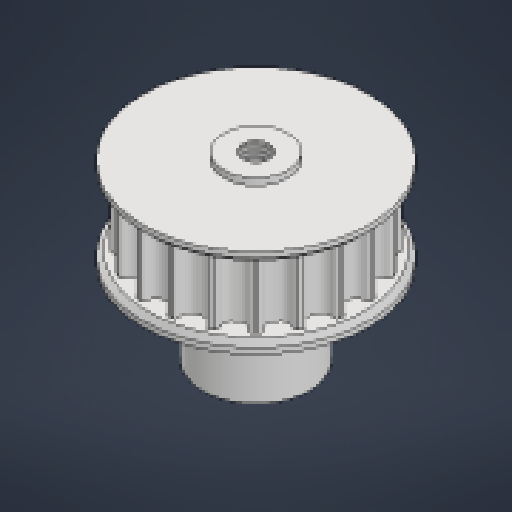
# Autodesk Inventor part: 3DPRINT,ROLLER,PLUG,SHORT
Saved by Autodesk Inventor 2026.1 (Build 301233020, 233B)
## iProperties
Created: 2026-03-30
Part Number: 3DPRINT,ROLLER,PLUG,SHORT
Material: Generic
Document SubType Name: Modeling
Designer: Owen L
Density: 1 g/cm^3
Appearance: Default
Author: Owen L
Autodesk Inventor part; units mm, degrees
(part 1 of 2)
ref_plane "YZ Plane" through (0, 0, 0) normal (1, 0, 0) x (0, 1, 0)
ref_plane "XZ Plane" through (0, 0, 0) normal (0, 1, 0) x (-1, 0, 0)
ref_plane "XY Plane" through (0, 0, 0) normal (0, 0, 1) x (1, 0, 0)
sketch "Sketch1" plane through (0, 0, 0) normal (0, 1, 0) x (-1, 0, 0)
  arc A0 (15.108, -2.6737) -> (15.1947, -2.1258) centre (0, 0) ccw
  spline S0 degree 3 poles (15.108, -2.6737) (15.0887, -2.737) (15.0572, -2.7959) (14.9734, -2.8984) (14.922, -2.941) (14.8056, -3.0039) (14.7419, -3.0237) (14.6027, -3.0386) (14.545, -3.0287) (14.2674, -2.9716) (14.0596, -2.9092) (13.6157, -2.9838) (13.4596, -3.0427) (13.1787, -3.2171) (13.0566, -3.3308) (12.8434, -3.6259) (12.7944, -3.773) (12.6632, -4.1825) (12.5425, -4.4508) (12.5133, -4.8985) (12.5344, -5.0632) (12.6389, -5.3764) (12.7214, -5.5216) (12.91, -5.7403) (13.0253, -5.8538) (13.397, -6.0406) (13.5567, -6.0705) (13.7265, -6.2474) (13.7625, -6.3037) (13.8087, -6.4211) (13.8206, -6.4805) (13.8232, -6.6006) (13.8138, -6.6604) (13.7941, -6.7172) knots 0 0 0 0 0.019863 0.019863 0.03972 0.03972 0.059573 0.059573 0.081705 0.081705 0.153115 0.153115 0.194508 0.194508 0.235922 0.235922 0.285548 0.285548 0.382717 0.382717 0.438735 0.438735 0.494976 0.494976 0.536961 0.536961 0.576712 0.576712 0.591396 0.591396 0.604738 0.604738 0.618079 0.618079 0.618079 0.618079
  line L0 (15.108, -2.6737) -> (15.0887, -2.737) construction
  line L1 (15.0887, -2.737) -> (15.0572, -2.7959) construction
  line L2 (15.0572, -2.7959) -> (14.9734, -2.8984) construction
  line L3 (14.9734, -2.8984) -> (14.922, -2.941) construction
  line L4 (14.922, -2.941) -> (14.8056, -3.0039) construction
  line L5 (14.8056, -3.0039) -> (14.7419, -3.0237) construction
  line L6 (14.7419, -3.0237) -> (14.6027, -3.0386) construction
  line L7 (14.6027, -3.0386) -> (14.545, -3.0287) construction
  line L8 (14.545, -3.0287) -> (14.2674, -2.9716) construction
  line L9 (14.2674, -2.9716) -> (14.0596, -2.9092) construction
  line L10 (14.0596, -2.9092) -> (13.6157, -2.9838) construction
  line L11 (13.6157, -2.9838) -> (13.4596, -3.0427) construction
  line L12 (13.4596, -3.0427) -> (13.1787, -3.2171) construction
  line L13 (13.1787, -3.2171) -> (13.0566, -3.3308) construction
  line L14 (13.0566, -3.3308) -> (12.8434, -3.6259) construction
  line L15 (12.8434, -3.6259) -> (12.7944, -3.773) construction
  line L16 (12.7944, -3.773) -> (12.6632, -4.1825) construction
  line L17 (12.6632, -4.1825) -> (12.5425, -4.4508) construction
  line L18 (12.5425, -4.4508) -> (12.5133, -4.8985) construction
  line L19 (12.5133, -4.8985) -> (12.5344, -5.0632) construction
  line L20 (12.5344, -5.0632) -> (12.6389, -5.3764) construction
  line L21 (12.6389, -5.3764) -> (12.7214, -5.5216) construction
  line L22 (12.7214, -5.5216) -> (12.91, -5.7403) construction
  line L23 (12.91, -5.7403) -> (13.0253, -5.8538) construction
  line L24 (13.0253, -5.8538) -> (13.397, -6.0406) construction
  line L25 (13.397, -6.0406) -> (13.5567, -6.0705) construction
  line L26 (13.5567, -6.0705) -> (13.7265, -6.2474) construction
  line L27 (13.7265, -6.2474) -> (13.7625, -6.3037) construction
  line L28 (13.7625, -6.3037) -> (13.8087, -6.4211) construction
  line L29 (13.8087, -6.4211) -> (13.8206, -6.4805) construction
  line L30 (13.8206, -6.4805) -> (13.8232, -6.6006) construction
  line L31 (13.8232, -6.6006) -> (13.8138, -6.6604) construction
  line L32 (13.8138, -6.6604) -> (13.7941, -6.7172) construction
  arc A1 (13.5423, -7.2114) -> (13.7941, -6.7172) centre (0, 0) ccw
  spline S1 degree 3 poles (13.5423, -7.2114) (13.5044, -7.2657) (13.4563, -7.312) (13.3449, -7.3836) (13.2828, -7.4082) (13.1527, -7.4321) (13.0859, -7.4312) (12.949, -7.4024) (12.8972, -7.3751) (12.6509, -7.235) (12.4725, -7.1115) (12.0272, -7.0452) (11.8606, -7.053) (11.5395, -7.1321) (11.3883, -7.2025) (11.0944, -7.4173) (11.0023, -7.542) (10.751, -7.8909) (10.5533, -8.1088) (10.3871, -8.5256) (10.3563, -8.6887) (10.3589, -9.0189) (10.3925, -9.1825) (10.5043, -9.4488) (10.5789, -9.5924) (10.8746, -9.8848) (11.0174, -9.9626) (11.1241, -10.1834) (11.1409, -10.248) (11.1486, -10.374) (11.1416, -10.4341) (11.1069, -10.5491) (11.0795, -10.6031) (11.0433, -10.6511) knots 0 0 0 0 0.019863 0.019863 0.03972 0.03972 0.059573 0.059573 0.081705 0.081705 0.153115 0.153115 0.194508 0.194508 0.235922 0.235922 0.285548 0.285548 0.382717 0.382717 0.438735 0.438735 0.494976 0.494976 0.536961 0.536961 0.576712 0.576712 0.591396 0.591396 0.604738 0.604738 0.618079 0.618079 0.618079 0.618079
  line L33 (13.5423, -7.2114) -> (13.5044, -7.2657) construction
  line L34 (13.5044, -7.2657) -> (13.4563, -7.312) construction
  line L35 (13.4563, -7.312) -> (13.3449, -7.3836) construction
  line L36 (13.3449, -7.3836) -> (13.2828, -7.4082) construction
  line L37 (13.2828, -7.4082) -> (13.1527, -7.4321) construction
  line L38 (13.1527, -7.4321) -> (13.0859, -7.4312) construction
  line L39 (13.0859, -7.4312) -> (12.949, -7.4024) construction
  line L40 (12.949, -7.4024) -> (12.8972, -7.3751) construction
  line L41 (12.8972, -7.3751) -> (12.6509, -7.235) construction
  line L42 (12.6509, -7.235) -> (12.4725, -7.1115) construction
  line L43 (12.4725, -7.1115) -> (12.0272, -7.0452) construction
  line L44 (12.0272, -7.0452) -> (11.8606, -7.053) construction
  line L45 (11.8606, -7.053) -> (11.5395, -7.1321) construction
  line L46 (11.5395, -7.1321) -> (11.3883, -7.2025) construction
  line L47 (11.3883, -7.2025) -> (11.0944, -7.4173) construction
  line L48 (11.0944, -7.4173) -> (11.0023, -7.542) construction
  line L49 (11.0023, -7.542) -> (10.751, -7.8909) construction
  line L50 (10.751, -7.8909) -> (10.5533, -8.1088) construction
  line L51 (10.5533, -8.1088) -> (10.3871, -8.5256) construction
  line L52 (10.3871, -8.5256) -> (10.3563, -8.6887) construction
  line L53 (10.3563, -8.6887) -> (10.3589, -9.0189) construction
  line L54 (10.3589, -9.0189) -> (10.3925, -9.1825) construction
  line L55 (10.3925, -9.1825) -> (10.5043, -9.4488) construction
  line L56 (10.5043, -9.4488) -> (10.5789, -9.5924) construction
  line L57 (10.5789, -9.5924) -> (10.8746, -9.8848) construction
  line L58 (10.8746, -9.8848) -> (11.0174, -9.9626) construction
  line L59 (11.0174, -9.9626) -> (11.1241, -10.1834) construction
  line L60 (11.1241, -10.1834) -> (11.1409, -10.248) construction
  line L61 (11.1409, -10.248) -> (11.1486, -10.374) construction
  line L62 (11.1486, -10.374) -> (11.1416, -10.4341) construction
  line L63 (11.1416, -10.4341) -> (11.1069, -10.5491) construction
  line L64 (11.1069, -10.5491) -> (11.0795, -10.6031) construction
  line L65 (11.0795, -10.6031) -> (11.0433, -10.6511) construction
  arc A2 (10.6511, -11.0433) -> (11.0433, -10.6511) centre (0, 0) ccw
  spline S2 degree 3 poles (10.6511, -11.0433) (10.5982, -11.0832) (10.5381, -11.1124) (10.4101, -11.146) (10.3435, -11.1502) (10.2123, -11.1327) (10.1491, -11.1113) (10.0277, -11.0415) (9.987, -10.9996) (9.7959, -10.7903) (9.6645, -10.6176) (9.2615, -10.417) (9.1006, -10.373) (8.7708, -10.3489) (8.6052, -10.3692) (8.2593, -10.4826) (8.1332, -10.5728) (7.7864, -10.8269) (7.531, -10.9731) (7.2442, -11.3181) (7.1645, -11.4638) (7.0649, -11.7786) (7.0464, -11.9445) (7.0704, -12.2323) (7.0969, -12.3919) (7.2878, -12.7615) (7.3995, -12.8796) (7.4328, -13.1225) (7.4289, -13.1891) (7.3972, -13.3113) (7.372, -13.3664) (7.3034, -13.465) (7.2607, -13.5079) (7.2114, -13.5423) knots 0 0 0 0 0.019863 0.019863 0.03972 0.03972 0.059573 0.059573 0.081705 0.081705 0.153115 0.153115 0.194508 0.194508 0.235922 0.235922 0.285548 0.285548 0.382717 0.382717 0.438735 0.438735 0.494976 0.494976 0.536961 0.536961 0.576712 0.576712 0.591396 0.591396 0.604738 0.604738 0.618079 0.618079 0.618079 0.618079
  line L66 (10.6511, -11.0433) -> (10.5982, -11.0832) construction
  line L67 (10.5982, -11.0832) -> (10.5381, -11.1124) construction
  line L68 (10.5381, -11.1124) -> (10.4101, -11.146) construction
  line L69 (10.4101, -11.146) -> (10.3435, -11.1502) construction
  line L70 (10.3435, -11.1502) -> (10.2123, -11.1327) construction
  line L71 (10.2123, -11.1327) -> (10.1491, -11.1113) construction
  line L72 (10.1491, -11.1113) -> (10.0277, -11.0415) construction
  line L73 (10.0277, -11.0415) -> (9.987, -10.9996) construction
  line L74 (9.987, -10.9996) -> (9.7959, -10.7903) construction
  line L75 (9.7959, -10.7903) -> (9.6645, -10.6176) construction
  line L76 (9.6645, -10.6176) -> (9.2615, -10.417) construction
  line L77 (9.2615, -10.417) -> (9.1006, -10.373) construction
  line L78 (9.1006, -10.373) -> (8.7708, -10.3489) construction
  line L79 (8.7708, -10.3489) -> (8.6052, -10.3692) construction
  line L80 (8.6052, -10.3692) -> (8.2593, -10.4826) construction
  line L81 (8.2593, -10.4826) -> (8.1332, -10.5728) construction
  line L82 (8.1332, -10.5728) -> (7.7864, -10.8269) construction
  line L83 (7.7864, -10.8269) -> (7.531, -10.9731) construction
  line L84 (7.531, -10.9731) -> (7.2442, -11.3181) construction
  line L85 (7.2442, -11.3181) -> (7.1645, -11.4638) construction
  line L86 (7.1645, -11.4638) -> (7.0649, -11.7786) construction
  line L87 (7.0649, -11.7786) -> (7.0464, -11.9445) construction
  line L88 (7.0464, -11.9445) -> (7.0704, -12.2323) construction
  line L89 (7.0704, -12.2323) -> (7.0969, -12.3919) construction
  line L90 (7.0969, -12.3919) -> (7.2878, -12.7615) construction
  line L91 (7.2878, -12.7615) -> (7.3995, -12.8796) construction
  line L92 (7.3995, -12.8796) -> (7.4328, -13.1225) construction
  line L93 (7.4328, -13.1225) -> (7.4289, -13.1891) construction
  line L94 (7.4289, -13.1891) -> (7.3972, -13.3113) construction
  line L95 (7.3972, -13.3113) -> (7.372, -13.3664) construction
  line L96 (7.372, -13.3664) -> (7.3034, -13.465) construction
  line L97 (7.3034, -13.465) -> (7.2607, -13.5079) construction
  line L98 (7.2607, -13.5079) -> (7.2114, -13.5423) construction
  arc A3 (6.7172, -13.7941) -> (7.2114, -13.5423) centre (0, 0) ccw
  spline S3 degree 3 poles (6.7172, -13.7941) (6.6546, -13.8158) (6.5884, -13.8249) (6.4563, -13.8174) (6.3916, -13.8008) (6.2723, -13.7436) (6.2188, -13.7037) (6.1249, -13.5999) (6.0991, -13.5474) (5.9821, -13.2893) (5.9105, -13.0845) (5.5892, -12.7691) (5.4498, -12.6775) (5.1435, -12.5527) (4.9798, -12.5209) (4.6158, -12.5218) (4.468, -12.5686) (4.0596, -12.7031) (3.7715, -12.7632) (3.3921, -13.0028) (3.2713, -13.1166) (3.0794, -13.3853) (3.0104, -13.5374) (2.9443, -13.8185) (2.9203, -13.9785) (2.9876, -14.3889) (3.0573, -14.5358) (3.0139, -14.7771) (2.9896, -14.8393) (2.9218, -14.9457) (2.8807, -14.9902) (2.7851, -15.0629) (2.7312, -15.0904) (2.6737, -15.108) knots 0 0 0 0 0.019863 0.019863 0.03972 0.03972 0.059573 0.059573 0.081705 0.081705 0.153115 0.153115 0.194508 0.194508 0.235922 0.235922 0.285548 0.285548 0.382717 0.382717 0.438735 0.438735 0.494976 0.494976 0.536961 0.536961 0.576712 0.576712 0.591396 0.591396 0.604738 0.604738 0.618079 0.618079 0.618079 0.618079
  line L99 (6.7172, -13.7941) -> (6.6546, -13.8158) construction
  line L100 (6.6546, -13.8158) -> (6.5884, -13.8249) construction
  line L101 (6.5884, -13.8249) -> (6.4563, -13.8174) construction
  line L102 (6.4563, -13.8174) -> (6.3916, -13.8008) construction
  line L103 (6.3916, -13.8008) -> (6.2723, -13.7436) construction
  line L104 (6.2723, -13.7436) -> (6.2188, -13.7037) construction
  line L105 (6.2188, -13.7037) -> (6.1249, -13.5999) construction
  line L106 (6.1249, -13.5999) -> (6.0991, -13.5474) construction
  line L107 (6.0991, -13.5474) -> (5.9821, -13.2893) construction
  line L108 (5.9821, -13.2893) -> (5.9105, -13.0845) construction
  line L109 (5.9105, -13.0845) -> (5.5892, -12.7691) construction
  line L110 (5.5892, -12.7691) -> (5.4498, -12.6775) construction
  line L111 (5.4498, -12.6775) -> (5.1435, -12.5527) construction
  line L112 (5.1435, -12.5527) -> (4.9798, -12.5209) construction
  line L113 (4.9798, -12.5209) -> (4.6158, -12.5218) construction
  line L114 (4.6158, -12.5218) -> (4.468, -12.5686) construction
  line L115 (4.468, -12.5686) -> (4.0596, -12.7031) construction
  line L116 (4.0596, -12.7031) -> (3.7715, -12.7632) construction
  line L117 (3.7715, -12.7632) -> (3.3921, -13.0028) construction
  line L118 (3.3921, -13.0028) -> (3.2713, -13.1166) construction
  line L119 (3.2713, -13.1166) -> (3.0794, -13.3853) construction
  line L120 (3.0794, -13.3853) -> (3.0104, -13.5374) construction
  line L121 (3.0104, -13.5374) -> (2.9443, -13.8185) construction
  line L122 (2.9443, -13.8185) -> (2.9203, -13.9785) construction
  line L123 (2.9203, -13.9785) -> (2.9876, -14.3889) construction
  line L124 (2.9876, -14.3889) -> (3.0573, -14.5358) construction
  line L125 (3.0573, -14.5358) -> (3.0139, -14.7771) construction
  line L126 (3.0139, -14.7771) -> (2.9896, -14.8393) construction
  line L127 (2.9896, -14.8393) -> (2.9218, -14.9457) construction
  line L128 (2.9218, -14.9457) -> (2.8807, -14.9902) construction
  line L129 (2.8807, -14.9902) -> (2.7851, -15.0629) construction
  line L130 (2.7851, -15.0629) -> (2.7312, -15.0904) construction
  line L131 (2.7312, -15.0904) -> (2.6737, -15.108) construction
  arc A4 (2.1258, -15.1947) -> (2.6737, -15.108) centre (0, 0) ccw
  spline S4 degree 3 poles (2.1258, -15.1947) (2.0596, -15.196) (1.9938, -15.1842) (1.8705, -15.1362) (1.8141, -15.1004) (1.7183, -15.0092) (1.6797, -14.9547) (1.6226, -14.827) (1.6142, -14.7691) (1.5827, -14.4874) (1.5779, -14.2705) (1.3697, -13.8713) (1.2655, -13.7411) (1.0128, -13.5278) (0.8669, -13.4469) (0.5204, -13.3353) (0.3654, -13.3341) (-0.0646, -13.3359) (-0.3571, -13.304) (-0.792, -13.4146) (-0.942, -13.4856) (-1.2076, -13.6817) (-1.3202, -13.8051) (-1.4699, -14.052) (-1.5423, -14.1967) (-1.605, -14.6079) (-1.5841, -14.7691) (-1.7, -14.9852) (-1.7423, -15.0368) (-1.8397, -15.1171) (-1.8925, -15.1468) (-2.0059, -15.1863) (-2.0657, -15.1958) (-2.1258, -15.1947) knots 0 0 0 0 0.019863 0.019863 0.03972 0.03972 0.059573 0.059573 0.081705 0.081705 0.153115 0.153115 0.194508 0.194508 0.235922 0.235922 0.285548 0.285548 0.382717 0.382717 0.438735 0.438735 0.494976 0.494976 0.536961 0.536961 0.576712 0.576712 0.591396 0.591396 0.604738 0.604738 0.618079 0.618079 0.618079 0.618079
  line L132 (2.1258, -15.1947) -> (2.0596, -15.196) construction
  line L133 (2.0596, -15.196) -> (1.9938, -15.1842) construction
  line L134 (1.9938, -15.1842) -> (1.8705, -15.1362) construction
  line L135 (1.8705, -15.1362) -> (1.8141, -15.1004) construction
  line L136 (1.8141, -15.1004) -> (1.7183, -15.0092) construction
  line L137 (1.7183, -15.0092) -> (1.6797, -14.9547) construction
  line L138 (1.6797, -14.9547) -> (1.6226, -14.827) construction
  line L139 (1.6226, -14.827) -> (1.6142, -14.7691) construction
  line L140 (1.6142, -14.7691) -> (1.5827, -14.4874) construction
  line L141 (1.5827, -14.4874) -> (1.5779, -14.2705) construction
  line L142 (1.5779, -14.2705) -> (1.3697, -13.8713) construction
  line L143 (1.3697, -13.8713) -> (1.2655, -13.7411) construction
  line L144 (1.2655, -13.7411) -> (1.0128, -13.5278) construction
  line L145 (1.0128, -13.5278) -> (0.8669, -13.4469) construction
  line L146 (0.8669, -13.4469) -> (0.5204, -13.3353) construction
  line L147 (0.5204, -13.3353) -> (0.3654, -13.3341) construction
  line L148 (0.3654, -13.3341) -> (-0.0646, -13.3359) construction
  line L149 (-0.0646, -13.3359) -> (-0.3571, -13.304) construction
  line L150 (-0.3571, -13.304) -> (-0.792, -13.4146) construction
  line L151 (-0.792, -13.4146) -> (-0.942, -13.4856) construction
  line L152 (-0.942, -13.4856) -> (-1.2076, -13.6817) construction
  line L153 (-1.2076, -13.6817) -> (-1.3202, -13.8051) construction
  line L154 (-1.3202, -13.8051) -> (-1.4699, -14.052) construction
  line L155 (-1.4699, -14.052) -> (-1.5423, -14.1967) construction
  line L156 (-1.5423, -14.1967) -> (-1.605, -14.6079) construction
  line L157 (-1.605, -14.6079) -> (-1.5841, -14.7691) construction
  line L158 (-1.5841, -14.7691) -> (-1.7, -14.9852) construction
  line L159 (-1.7, -14.9852) -> (-1.7423, -15.0368) construction
  line L160 (-1.7423, -15.0368) -> (-1.8397, -15.1171) construction
  line L161 (-1.8397, -15.1171) -> (-1.8925, -15.1468) construction
  line L162 (-1.8925, -15.1468) -> (-2.0059, -15.1863) construction
  line L163 (-2.0059, -15.1863) -> (-2.0657, -15.1958) construction
  line L164 (-2.0657, -15.1958) -> (-2.1258, -15.1947) construction
  arc A5 (-2.6737, -15.108) -> (-2.1258, -15.1947) centre (0, 0) ccw
  spline S5 degree 3 poles (-2.6737, -15.108) (-2.737, -15.0887) (-2.7959, -15.0572) (-2.8984, -14.9734) (-2.941, -14.922) (-3.0039, -14.8056) (-3.0237, -14.7419) (-3.0386, -14.6027) (-3.0287, -14.545) (-2.9716, -14.2674) (-2.9092, -14.0596) (-2.9838, -13.6157) (-3.0427, -13.4596) (-3.2171, -13.1787) (-3.3308, -13.0566) (-3.6259, -12.8434) (-3.773, -12.7944) (-4.1825, -12.6632) (-4.4508, -12.5425) (-4.8985, -12.5133) (-5.0632, -12.5344) (-5.3764, -12.6389) (-5.5216, -12.7214) (-5.7403, -12.91) (-5.8538, -13.0253) (-6.0406, -13.397) (-6.0705, -13.5567) (-6.2474, -13.7265) (-6.3037, -13.7625) (-6.4211, -13.8087) (-6.4805, -13.8206) (-6.6006, -13.8232) (-6.6604, -13.8138) (-6.7172, -13.7941) knots 0 0 0 0 0.019863 0.019863 0.03972 0.03972 0.059573 0.059573 0.081705 0.081705 0.153115 0.153115 0.194508 0.194508 0.235922 0.235922 0.285548 0.285548 0.382717 0.382717 0.438735 0.438735 0.494976 0.494976 0.536961 0.536961 0.576712 0.576712 0.591396 0.591396 0.604738 0.604738 0.618079 0.618079 0.618079 0.618079
  line L165 (-2.6737, -15.108) -> (-2.737, -15.0887) construction
  line L166 (-2.737, -15.0887) -> (-2.7959, -15.0572) construction
  line L167 (-2.7959, -15.0572) -> (-2.8984, -14.9734) construction
  line L168 (-2.8984, -14.9734) -> (-2.941, -14.922) construction
  line L169 (-2.941, -14.922) -> (-3.0039, -14.8056) construction
  line L170 (-3.0039, -14.8056) -> (-3.0237, -14.7419) construction
  line L171 (-3.0237, -14.7419) -> (-3.0386, -14.6027) construction
  line L172 (-3.0386, -14.6027) -> (-3.0287, -14.545) construction
  line L173 (-3.0287, -14.545) -> (-2.9716, -14.2674) construction
  line L174 (-2.9716, -14.2674) -> (-2.9092, -14.0596) construction
  line L175 (-2.9092, -14.0596) -> (-2.9838, -13.6157) construction
  line L176 (-2.9838, -13.6157) -> (-3.0427, -13.4596) construction
  line L177 (-3.0427, -13.4596) -> (-3.2171, -13.1787) construction
  line L178 (-3.2171, -13.1787) -> (-3.3308, -13.0566) construction
  line L179 (-3.3308, -13.0566) -> (-3.6259, -12.8434) construction
  line L180 (-3.6259, -12.8434) -> (-3.773, -12.7944) construction
  line L181 (-3.773, -12.7944) -> (-4.1825, -12.6632) construction
  line L182 (-4.1825, -12.6632) -> (-4.4508, -12.5425) construction
  line L183 (-4.4508, -12.5425) -> (-4.8985, -12.5133) construction
  line L184 (-4.8985, -12.5133) -> (-5.0632, -12.5344) construction
  line L185 (-5.0632, -12.5344) -> (-5.3764, -12.6389) construction
  line L186 (-5.3764, -12.6389) -> (-5.5216, -12.7214) construction
  line L187 (-5.5216, -12.7214) -> (-5.7403, -12.91) construction
  line L188 (-5.7403, -12.91) -> (-5.8538, -13.0253) construction
  line L189 (-5.8538, -13.0253) -> (-6.0406, -13.397) construction
  line L190 (-6.0406, -13.397) -> (-6.0705, -13.5567) construction
  line L191 (-6.0705, -13.5567) -> (-6.2474, -13.7265) construction
  line L192 (-6.2474, -13.7265) -> (-6.3037, -13.7625) construction
  line L193 (-6.3037, -13.7625) -> (-6.4211, -13.8087) construction
  line L194 (-6.4211, -13.8087) -> (-6.4805, -13.8206) construction
  line L195 (-6.4805, -13.8206) -> (-6.6006, -13.8232) construction
  line L196 (-6.6006, -13.8232) -> (-6.6604, -13.8138) construction
  line L197 (-6.6604, -13.8138) -> (-6.7172, -13.7941) construction
  arc A6 (-7.2114, -13.5423) -> (-6.7172, -13.7941) centre (0, 0) ccw
  spline S6 degree 3 poles (-7.2114, -13.5423) (-7.2657, -13.5044) (-7.312, -13.4563) (-7.3836, -13.3449) (-7.4082, -13.2828) (-7.4321, -13.1527) (-7.4312, -13.0859) (-7.4024, -12.949) (-7.3751, -12.8972) (-7.235, -12.6509) (-7.1115, -12.4725) (-7.0452, -12.0272) (-7.053, -11.8606) (-7.1321, -11.5395) (-7.2025, -11.3883) (-7.4173, -11.0944) (-7.542, -11.0023) (-7.8909, -10.751) (-8.1088, -10.5533) (-8.5256, -10.3871) (-8.6887, -10.3563) (-9.0189, -10.3589) (-9.1825, -10.3925) (-9.4488, -10.5043) (-9.5924, -10.5789) (-9.8848, -10.8746) (-9.9626, -11.0174) (-10.1834, -11.1241) (-10.248, -11.1409) (-10.374, -11.1486) (-10.4341, -11.1416) (-10.5491, -11.1069) (-10.6031, -11.0795) (-10.6511, -11.0433) knots 0 0 0 0 0.019863 0.019863 0.03972 0.03972 0.059573 0.059573 0.081705 0.081705 0.153115 0.153115 0.194508 0.194508 0.235922 0.235922 0.285548 0.285548 0.382717 0.382717 0.438735 0.438735 0.494976 0.494976 0.536961 0.536961 0.576712 0.576712 0.591396 0.591396 0.604738 0.604738 0.618079 0.618079 0.618079 0.618079
  line L198 (-7.2114, -13.5423) -> (-7.2657, -13.5044) construction
  line L199 (-7.2657, -13.5044) -> (-7.312, -13.4563) construction
  line L200 (-7.312, -13.4563) -> (-7.3836, -13.3449) construction
  line L201 (-7.3836, -13.3449) -> (-7.4082, -13.2828) construction
  line L202 (-7.4082, -13.2828) -> (-7.4321, -13.1527) construction
  line L203 (-7.4321, -13.1527) -> (-7.4312, -13.0859) construction
  line L204 (-7.4312, -13.0859) -> (-7.4024, -12.949) construction
  line L205 (-7.4024, -12.949) -> (-7.3751, -12.8972) construction
  line L206 (-7.3751, -12.8972) -> (-7.235, -12.6509) construction
  line L207 (-7.235, -12.6509) -> (-7.1115, -12.4725) construction
  line L208 (-7.1115, -12.4725) -> (-7.0452, -12.0272) construction
  line L209 (-7.0452, -12.0272) -> (-7.053, -11.8606) construction
  line L210 (-7.053, -11.8606) -> (-7.1321, -11.5395) construction
  line L211 (-7.1321, -11.5395) -> (-7.2025, -11.3883) construction
  line L212 (-7.2025, -11.3883) -> (-7.4173, -11.0944) construction
  line L213 (-7.4173, -11.0944) -> (-7.542, -11.0023) construction
  line L214 (-7.542, -11.0023) -> (-7.8909, -10.751) construction
  line L215 (-7.8909, -10.751) -> (-8.1088, -10.5533) construction
  line L216 (-8.1088, -10.5533) -> (-8.5256, -10.3871) construction
  line L217 (-8.5256, -10.3871) -> (-8.6887, -10.3563) construction
  line L218 (-8.6887, -10.3563) -> (-9.0189, -10.3589) construction
  line L219 (-9.0189, -10.3589) -> (-9.1825, -10.3925) construction
  line L220 (-9.1825, -10.3925) -> (-9.4488, -10.5043) construction
  line L221 (-9.4488, -10.5043) -> (-9.5924, -10.5789) construction
  line L222 (-9.5924, -10.5789) -> (-9.8848, -10.8746) construction
  line L223 (-9.8848, -10.8746) -> (-9.9626, -11.0174) construction
  line L224 (-9.9626, -11.0174) -> (-10.1834, -11.1241) construction
  line L225 (-10.1834, -11.1241) -> (-10.248, -11.1409) construction
  line L226 (-10.248, -11.1409) -> (-10.374, -11.1486) construction
  line L227 (-10.374, -11.1486) -> (-10.4341, -11.1416) construction
  line L228 (-10.4341, -11.1416) -> (-10.5491, -11.1069) construction
  line L229 (-10.5491, -11.1069) -> (-10.6031, -11.0795) construction
  line L230 (-10.6031, -11.0795) -> (-10.6511, -11.0433) construction
  arc A7 (-11.0433, -10.6511) -> (-10.6511, -11.0433) centre (0, 0) ccw
  spline S7 degree 3 poles (-11.0433, -10.6511) (-11.0832, -10.5982) (-11.1124, -10.5381) (-11.146, -10.4101) (-11.1502, -10.3435) (-11.1327, -10.2123) (-11.1113, -10.1491) (-11.0415, -10.0277) (-10.9996, -9.987) (-10.7903, -9.7959) (-10.6176, -9.6645) (-10.417, -9.2615) (-10.373, -9.1006) (-10.3489, -8.7708) (-10.3692, -8.6052) (-10.4826, -8.2593) (-10.5728, -8.1332) (-10.8269, -7.7864) (-10.9731, -7.531) (-11.3181, -7.2442) (-11.4638, -7.1645) (-11.7786, -7.0649) (-11.9445, -7.0464) (-12.2323, -7.0704) (-12.3919, -7.0969) (-12.7615, -7.2878) (-12.8796, -7.3995) (-13.1225, -7.4328) (-13.1891, -7.4289) (-13.3113, -7.3972) (-13.3664, -7.372) (-13.465, -7.3034) (-13.5079, -7.2607) (-13.5423, -7.2114) knots 0 0 0 0 0.019863 0.019863 0.03972 0.03972 0.059573 0.059573 0.081705 0.081705 0.153115 0.153115 0.194508 0.194508 0.235922 0.235922 0.285548 0.285548 0.382717 0.382717 0.438735 0.438735 0.494976 0.494976 0.536961 0.536961 0.576712 0.576712 0.591396 0.591396 0.604738 0.604738 0.618079 0.618079 0.618079 0.618079
  line L231 (-11.0433, -10.6511) -> (-11.0832, -10.5982) construction
  line L232 (-11.0832, -10.5982) -> (-11.1124, -10.5381) construction
  line L233 (-11.1124, -10.5381) -> (-11.146, -10.4101) construction
  line L234 (-11.146, -10.4101) -> (-11.1502, -10.3435) construction
  line L235 (-11.1502, -10.3435) -> (-11.1327, -10.2123) construction
  line L236 (-11.1327, -10.2123) -> (-11.1113, -10.1491) construction
  line L237 (-11.1113, -10.1491) -> (-11.0415, -10.0277) construction
  line L238 (-11.0415, -10.0277) -> (-10.9996, -9.987) construction
  line L239 (-10.9996, -9.987) -> (-10.7903, -9.7959) construction
  line L240 (-10.7903, -9.7959) -> (-10.6176, -9.6645) construction
  line L241 (-10.6176, -9.6645) -> (-10.417, -9.2615) construction
  line L242 (-10.417, -9.2615) -> (-10.373, -9.1006) construction
  line L243 (-10.373, -9.1006) -> (-10.3489, -8.7708) construction
  line L244 (-10.3489, -8.7708) -> (-10.3692, -8.6052) construction
  line L245 (-10.3692, -8.6052) -> (-10.4826, -8.2593) construction
  line L246 (-10.4826, -8.2593) -> (-10.5728, -8.1332) construction
  line L247 (-10.5728, -8.1332) -> (-10.8269, -7.7864) construction
  line L248 (-10.8269, -7.7864) -> (-10.9731, -7.531) construction
  line L249 (-10.9731, -7.531) -> (-11.3181, -7.2442) construction
  line L250 (-11.3181, -7.2442) -> (-11.4638, -7.1645) construction
  line L251 (-11.4638, -7.1645) -> (-11.7786, -7.0649) construction
  line L252 (-11.7786, -7.0649) -> (-11.9445, -7.0464) construction
  line L253 (-11.9445, -7.0464) -> (-12.2323, -7.0704) construction
  line L254 (-12.2323, -7.0704) -> (-12.3919, -7.0969) construction
  line L255 (-12.3919, -7.0969) -> (-12.7615, -7.2878) construction
  line L256 (-12.7615, -7.2878) -> (-12.8796, -7.3995) construction
  line L257 (-12.8796, -7.3995) -> (-13.1225, -7.4328) construction
  line L258 (-13.1225, -7.4328) -> (-13.1891, -7.4289) construction
  line L259 (-13.1891, -7.4289) -> (-13.3113, -7.3972) construction
  line L260 (-13.3113, -7.3972) -> (-13.3664, -7.372) construction
  line L261 (-13.3664, -7.372) -> (-13.465, -7.3034) construction
  line L262 (-13.465, -7.3034) -> (-13.5079, -7.2607) construction
  line L263 (-13.5079, -7.2607) -> (-13.5423, -7.2114) construction
  arc A8 (-13.7941, -6.7172) -> (-13.5423, -7.2114) centre (0, 0) ccw
  spline S8 degree 3 poles (-13.7941, -6.7172) (-13.8158, -6.6546) (-13.8249, -6.5884) (-13.8174, -6.4563) (-13.8008, -6.3916) (-13.7436, -6.2723) (-13.7037, -6.2188) (-13.5999, -6.1249) (-13.5474, -6.0991) (-13.2893, -5.9821) (-13.0845, -5.9105) (-12.7691, -5.5892) (-12.6775, -5.4498) (-12.5527, -5.1435) (-12.5209, -4.9798) (-12.5218, -4.6158) (-12.5686, -4.468) (-12.7031, -4.0596) (-12.7632, -3.7715) (-13.0028, -3.3921) (-13.1166, -3.2713) (-13.3853, -3.0794) (-13.5374, -3.0104) (-13.8185, -2.9443) (-13.9785, -2.9203) (-14.3889, -2.9876) (-14.5358, -3.0573) (-14.7771, -3.0139) (-14.8393, -2.9896) (-14.9457, -2.9218) (-14.9902, -2.8807) (-15.0629, -2.7851) (-15.0904, -2.7312) (-15.108, -2.6737) knots 0 0 0 0 0.019863 0.019863 0.03972 0.03972 0.059573 0.059573 0.081705 0.081705 0.153115 0.153115 0.194508 0.194508 0.235922 0.235922 0.285548 0.285548 0.382717 0.382717 0.438735 0.438735 0.494976 0.494976 0.536961 0.536961 0.576712 0.576712 0.591396 0.591396 0.604738 0.604738 0.618079 0.618079 0.618079 0.618079
  line L264 (-13.7941, -6.7172) -> (-13.8158, -6.6546) construction
  line L265 (-13.8158, -6.6546) -> (-13.8249, -6.5884) construction
  line L266 (-13.8249, -6.5884) -> (-13.8174, -6.4563) construction
  line L267 (-13.8174, -6.4563) -> (-13.8008, -6.3916) construction
  line L268 (-13.8008, -6.3916) -> (-13.7436, -6.2723) construction
  line L269 (-13.7436, -6.2723) -> (-13.7037, -6.2188) construction
  line L270 (-13.7037, -6.2188) -> (-13.5999, -6.1249) construction
  line L271 (-13.5999, -6.1249) -> (-13.5474, -6.0991) construction
  line L272 (-13.5474, -6.0991) -> (-13.2893, -5.9821) construction
  line L273 (-13.2893, -5.9821) -> (-13.0845, -5.9105) construction
  line L274 (-13.0845, -5.9105) -> (-12.7691, -5.5892) construction
  line L275 (-12.7691, -5.5892) -> (-12.6775, -5.4498) construction
  line L276 (-12.6775, -5.4498) -> (-12.5527, -5.1435) construction
  line L277 (-12.5527, -5.1435) -> (-12.5209, -4.9798) construction
  line L278 (-12.5209, -4.9798) -> (-12.5218, -4.6158) construction
  line L279 (-12.5218, -4.6158) -> (-12.5686, -4.468) construction
  line L280 (-12.5686, -4.468) -> (-12.7031, -4.0596) construction
  line L281 (-12.7031, -4.0596) -> (-12.7632, -3.7715) construction
  line L282 (-12.7632, -3.7715) -> (-13.0028, -3.3921) construction
  line L283 (-13.0028, -3.3921) -> (-13.1166, -3.2713) construction
  line L284 (-13.1166, -3.2713) -> (-13.3853, -3.0794) construction
  line L285 (-13.3853, -3.0794) -> (-13.5374, -3.0104) construction
  line L286 (-13.5374, -3.0104) -> (-13.8185, -2.9443) construction
  line L287 (-13.8185, -2.9443) -> (-13.9785, -2.9203) construction
  line L288 (-13.9785, -2.9203) -> (-14.3889, -2.9876) construction
  line L289 (-14.3889, -2.9876) -> (-14.5358, -3.0573) construction
  line L290 (-14.5358, -3.0573) -> (-14.7771, -3.0139) construction
  line L291 (-14.7771, -3.0139) -> (-14.8393, -2.9896) construction
  line L292 (-14.8393, -2.9896) -> (-14.9457, -2.9218) construction
  line L293 (-14.9457, -2.9218) -> (-14.9902, -2.8807) construction
  line L294 (-14.9902, -2.8807) -> (-15.0629, -2.7851) construction
  line L295 (-15.0629, -2.7851) -> (-15.0904, -2.7312) construction
  line L296 (-15.0904, -2.7312) -> (-15.108, -2.6737) construction
  arc A9 (-15.1947, -2.1258) -> (-15.108, -2.6737) centre (0, 0) ccw
  spline S9 degree 3 poles (-15.1947, -2.1258) (-15.196, -2.0596) (-15.1842, -1.9938) (-15.1362, -1.8705) (-15.1004, -1.8141) (-15.0092, -1.7183) (-14.9547, -1.6797) (-14.827, -1.6226) (-14.7691, -1.6142) (-14.4874, -1.5827) (-14.2705, -1.5779) (-13.8713, -1.3697) (-13.7411, -1.2655) (-13.5278, -1.0128) (-13.4469, -0.8669) (-13.3353, -0.5204) (-13.3341, -0.3654) (-13.3359, 0.0646) (-13.304, 0.3571) (-13.4146, 0.792) (-13.4856, 0.942) (-13.6817, 1.2076) (-13.8051, 1.3202) (-14.052, 1.4699) (-14.1967, 1.5423) (-14.6079, 1.605) (-14.7691, 1.5841) (-14.9852, 1.7) (-15.0368, 1.7423) (-15.1171, 1.8397) (-15.1468, 1.8925) (-15.1863, 2.0059) (-15.1958, 2.0657) (-15.1947, 2.1258) knots 0 0 0 0 0.019863 0.019863 0.03972 0.03972 0.059573 0.059573 0.081705 0.081705 0.153115 0.153115 0.194508 0.194508 0.235922 0.235922 0.285548 0.285548 0.382717 0.382717 0.438735 0.438735 0.494976 0.494976 0.536961 0.536961 0.576712 0.576712 0.591396 0.591396 0.604738 0.604738 0.618079 0.618079 0.618079 0.618079
  line L297 (-15.1947, -2.1258) -> (-15.196, -2.0596) construction
  line L298 (-15.196, -2.0596) -> (-15.1842, -1.9938) construction
  line L299 (-15.1842, -1.9938) -> (-15.1362, -1.8705) construction
  line L300 (-15.1362, -1.8705) -> (-15.1004, -1.8141) construction
  line L301 (-15.1004, -1.8141) -> (-15.0092, -1.7183) construction
  line L302 (-15.0092, -1.7183) -> (-14.9547, -1.6797) construction
  line L303 (-14.9547, -1.6797) -> (-14.827, -1.6226) construction
  line L304 (-14.827, -1.6226) -> (-14.7691, -1.6142) construction
  line L305 (-14.7691, -1.6142) -> (-14.4874, -1.5827) construction
  line L306 (-14.4874, -1.5827) -> (-14.2705, -1.5779) construction
  line L307 (-14.2705, -1.5779) -> (-13.8713, -1.3697) construction
  line L308 (-13.8713, -1.3697) -> (-13.7411, -1.2655) construction
  line L309 (-13.7411, -1.2655) -> (-13.5278, -1.0128) construction
  line L310 (-13.5278, -1.0128) -> (-13.4469, -0.8669) construction
  line L311 (-13.4469, -0.8669) -> (-13.3353, -0.5204) construction
  line L312 (-13.3353, -0.5204) -> (-13.3341, -0.3654) construction
  line L313 (-13.3341, -0.3654) -> (-13.3359, 0.0646) construction
  line L314 (-13.3359, 0.0646) -> (-13.304, 0.3571) construction
  line L315 (-13.304, 0.3571) -> (-13.4146, 0.792) construction
  line L316 (-13.4146, 0.792) -> (-13.4856, 0.942) construction
  line L317 (-13.4856, 0.942) -> (-13.6817, 1.2076) construction
  line L318 (-13.6817, 1.2076) -> (-13.8051, 1.3202) construction
  line L319 (-13.8051, 1.3202) -> (-14.052, 1.4699) construction
  line L320 (-14.052, 1.4699) -> (-14.1967, 1.5423) construction
  line L321 (-14.1967, 1.5423) -> (-14.6079, 1.605) construction
  line L322 (-14.6079, 1.605) -> (-14.7691, 1.5841) construction
  line L323 (-14.7691, 1.5841) -> (-14.9852, 1.7) construction
  line L324 (-14.9852, 1.7) -> (-15.0368, 1.7423) construction
  line L325 (-15.0368, 1.7423) -> (-15.1171, 1.8397) construction
  line L326 (-15.1171, 1.8397) -> (-15.1468, 1.8925) construction
  line L327 (-15.1468, 1.8925) -> (-15.1863, 2.0059) construction
  line L328 (-15.1863, 2.0059) -> (-15.1958, 2.0657) construction
  line L329 (-15.1958, 2.0657) -> (-15.1947, 2.1258) construction
  arc A10 (-15.108, 2.6737) -> (-15.1947, 2.1258) centre (0, 0) ccw
  spline S10 degree 3 poles (-15.108, 2.6737) (-15.0887, 2.737) (-15.0572, 2.7959) (-14.9734, 2.8984) (-14.922, 2.941) (-14.8056, 3.0039) (-14.7419, 3.0237) (-14.6027, 3.0386) (-14.545, 3.0287) (-14.2674, 2.9716) (-14.0596, 2.9092) (-13.6157, 2.9838) (-13.4596, 3.0427) (-13.1787, 3.2171) (-13.0566, 3.3308) (-12.8434, 3.6259) (-12.7944, 3.773) (-12.6632, 4.1825) (-12.5425, 4.4508) (-12.5133, 4.8985) (-12.5344, 5.0632) (-12.6389, 5.3764) (-12.7214, 5.5216) (-12.91, 5.7403) (-13.0253, 5.8538) (-13.397, 6.0406) (-13.5567, 6.0705) (-13.7265, 6.2474) (-13.7625, 6.3037) (-13.8087, 6.4211) (-13.8206, 6.4805) (-13.8232, 6.6006) (-13.8138, 6.6604) (-13.7941, 6.7172) knots 0 0 0 0 0.019863 0.019863 0.03972 0.03972 0.059573 0.059573 0.081705 0.081705 0.153115 0.153115 0.194508 0.194508 0.235922 0.235922 0.285548 0.285548 0.382717 0.382717 0.438735 0.438735 0.494976 0.494976 0.536961 0.536961 0.576712 0.576712 0.591396 0.591396 0.604738 0.604738 0.618079 0.618079 0.618079 0.618079
  line L330 (-15.108, 2.6737) -> (-15.0887, 2.737) construction
  line L331 (-15.0887, 2.737) -> (-15.0572, 2.7959) construction
  line L332 (-15.0572, 2.7959) -> (-14.9734, 2.8984) construction
  line L333 (-14.9734, 2.8984) -> (-14.922, 2.941) construction
  line L334 (-14.922, 2.941) -> (-14.8056, 3.0039) construction
  line L335 (-14.8056, 3.0039) -> (-14.7419, 3.0237) construction
  line L336 (-14.7419, 3.0237) -> (-14.6027, 3.0386) construction
  line L337 (-14.6027, 3.0386) -> (-14.545, 3.0287) construction
  line L338 (-14.545, 3.0287) -> (-14.2674, 2.9716) construction
  line L339 (-14.2674, 2.9716) -> (-14.0596, 2.9092) construction
  line L340 (-14.0596, 2.9092) -> (-13.6157, 2.9838) construction
  line L341 (-13.6157, 2.9838) -> (-13.4596, 3.0427) construction
  line L342 (-13.4596, 3.0427) -> (-13.1787, 3.2171) construction
  line L343 (-13.1787, 3.2171) -> (-13.0566, 3.3308) construction
  line L344 (-13.0566, 3.3308) -> (-12.8434, 3.6259) construction
  line L345 (-12.8434, 3.6259) -> (-12.7944, 3.773) construction
  line L346 (-12.7944, 3.773) -> (-12.6632, 4.1825) construction
  line L347 (-12.6632, 4.1825) -> (-12.5425, 4.4508) construction
  line L348 (-12.5425, 4.4508) -> (-12.5133, 4.8985) construction
  line L349 (-12.5133, 4.8985) -> (-12.5344, 5.0632) construction
  line L350 (-12.5344, 5.0632) -> (-12.6389, 5.3764) construction
  line L351 (-12.6389, 5.3764) -> (-12.7214, 5.5216) construction
  line L352 (-12.7214, 5.5216) -> (-12.91, 5.7403) construction
  line L353 (-12.91, 5.7403) -> (-13.0253, 5.8538) construction
  line L354 (-13.0253, 5.8538) -> (-13.397, 6.0406) construction
  line L355 (-13.397, 6.0406) -> (-13.5567, 6.0705) construction
  line L356 (-13.5567, 6.0705) -> (-13.7265, 6.2474) construction
  line L357 (-13.7265, 6.2474) -> (-13.7625, 6.3037) construction
  line L358 (-13.7625, 6.3037) -> (-13.8087, 6.4211) construction
  line L359 (-13.8087, 6.4211) -> (-13.8206, 6.4805) construction
  line L360 (-13.8206, 6.4805) -> (-13.8232, 6.6006) construction
  line L361 (-13.8232, 6.6006) -> (-13.8138, 6.6604) construction
  line L362 (-13.8138, 6.6604) -> (-13.7941, 6.7172) construction
  arc A11 (-13.5423, 7.2114) -> (-13.7941, 6.7172) centre (0, 0) ccw
  spline S11 degree 3 poles (-13.5423, 7.2114) (-13.5044, 7.2657) (-13.4563, 7.312) (-13.3449, 7.3836) (-13.2828, 7.4082) (-13.1527, 7.4321) (-13.0859, 7.4312) (-12.949, 7.4024) (-12.8972, 7.3751) (-12.6509, 7.235) (-12.4725, 7.1115) (-12.0272, 7.0452) (-11.8606, 7.053) (-11.5395, 7.1321) (-11.3883, 7.2025) (-11.0944, 7.4173) (-11.0023, 7.542) (-10.751, 7.8909) (-10.5533, 8.1088) (-10.3871, 8.5256) (-10.3563, 8.6887) (-10.3589, 9.0189) (-10.3925, 9.1825) (-10.5043, 9.4488) (-10.5789, 9.5924) (-10.8746, 9.8848) (-11.0174, 9.9626) (-11.1241, 10.1834) (-11.1409, 10.248) (-11.1486, 10.374) (-11.1416, 10.4341) (-11.1069, 10.5491) (-11.0795, 10.6031) (-11.0433, 10.6511) knots 0 0 0 0 0.019863 0.019863 0.03972 0.03972 0.059573 0.059573 0.081705 0.081705 0.153115 0.153115 0.194508 0.194508 0.235922 0.235922 0.285548 0.285548 0.382717 0.382717 0.438735 0.438735 0.494976 0.494976 0.536961 0.536961 0.576712 0.576712 0.591396 0.591396 0.604738 0.604738 0.618079 0.618079 0.618079 0.618079
  line L363 (-13.5423, 7.2114) -> (-13.5044, 7.2657) construction
  line L364 (-13.5044, 7.2657) -> (-13.4563, 7.312) construction
  line L365 (-13.4563, 7.312) -> (-13.3449, 7.3836) construction
  line L366 (-13.3449, 7.3836) -> (-13.2828, 7.4082) construction
  line L367 (-13.2828, 7.4082) -> (-13.1527, 7.4321) construction
  line L368 (-13.1527, 7.4321) -> (-13.0859, 7.4312) construction
  line L369 (-13.0859, 7.4312) -> (-12.949, 7.4024) construction
  line L370 (-12.949, 7.4024) -> (-12.8972, 7.3751) construction
  line L371 (-12.8972, 7.3751) -> (-12.6509, 7.235) construction
  line L372 (-12.6509, 7.235) -> (-12.4725, 7.1115) construction
  line L373 (-12.4725, 7.1115) -> (-12.0272, 7.0452) construction
  line L374 (-12.0272, 7.0452) -> (-11.8606, 7.053) construction
  line L375 (-11.8606, 7.053) -> (-11.5395, 7.1321) construction
  line L376 (-11.5395, 7.1321) -> (-11.3883, 7.2025) construction
  line L377 (-11.3883, 7.2025) -> (-11.0944, 7.4173) construction
  line L378 (-11.0944, 7.4173) -> (-11.0023, 7.542) construction
  line L379 (-11.0023, 7.542) -> (-10.751, 7.8909) construction
  line L380 (-10.751, 7.8909) -> (-10.5533, 8.1088) construction
  line L381 (-10.5533, 8.1088) -> (-10.3871, 8.5256) construction
  line L382 (-10.3871, 8.5256) -> (-10.3563, 8.6887) construction
  line L383 (-10.3563, 8.6887) -> (-10.3589, 9.0189) construction
  line L384 (-10.3589, 9.0189) -> (-10.3925, 9.1825) construction
  line L385 (-10.3925, 9.1825) -> (-10.5043, 9.4488) construction
  line L386 (-10.5043, 9.4488) -> (-10.5789, 9.5924) construction
  line L387 (-10.5789, 9.5924) -> (-10.8746, 9.8848) construction
  line L388 (-10.8746, 9.8848) -> (-11.0174, 9.9626) construction
  line L389 (-11.0174, 9.9626) -> (-11.1241, 10.1834) construction
  line L390 (-11.1241, 10.1834) -> (-11.1409, 10.248) construction
  line L391 (-11.1409, 10.248) -> (-11.1486, 10.374) construction
  line L392 (-11.1486, 10.374) -> (-11.1416, 10.4341) construction
  line L393 (-11.1416, 10.4341) -> (-11.1069, 10.5491) construction
  line L394 (-11.1069, 10.5491) -> (-11.0795, 10.6031) construction
  line L395 (-11.0795, 10.6031) -> (-11.0433, 10.6511) construction
  arc A12 (-10.6511, 11.0433) -> (-11.0433, 10.6511) centre (0, 0) ccw
  spline S12 degree 3 poles (-10.6511, 11.0433) (-10.5982, 11.0832) (-10.5381, 11.1124) (-10.4101, 11.146) (-10.3435, 11.1502) (-10.2123, 11.1327) (-10.1491, 11.1113) (-10.0277, 11.0415) (-9.987, 10.9996) (-9.7959, 10.7903) (-9.6645, 10.6176) (-9.2615, 10.417) (-9.1006, 10.373) (-8.7708, 10.3489) (-8.6052, 10.3692) (-8.2593, 10.4826) (-8.1332, 10.5728) (-7.7864, 10.8269) (-7.531, 10.9731) (-7.2442, 11.3181) (-7.1645, 11.4638) (-7.0649, 11.7786) (-7.0464, 11.9445) (-7.0704, 12.2323) (-7.0969, 12.3919) (-7.2878, 12.7615) (-7.3995, 12.8796) (-7.4328, 13.1225) (-7.4289, 13.1891) (-7.3972, 13.3113) (-7.372, 13.3664) (-7.3034, 13.465) (-7.2607, 13.5079) (-7.2114, 13.5423) knots 0 0 0 0 0.019863 0.019863 0.03972 0.03972 0.059573 0.059573 0.081705 0.081705 0.153115 0.153115 0.194508 0.194508 0.235922 0.235922 0.285548 0.285548 0.382717 0.382717 0.438735 0.438735 0.494976 0.494976 0.536961 0.536961 0.576712 0.576712 0.591396 0.591396 0.604738 0.604738 0.618079 0.618079 0.618079 0.618079
  line L396 (-10.6511, 11.0433) -> (-10.5982, 11.0832) construction
  line L397 (-10.5982, 11.0832) -> (-10.5381, 11.1124) construction
  line L398 (-10.5381, 11.1124) -> (-10.4101, 11.146) construction
  line L399 (-10.4101, 11.146) -> (-10.3435, 11.1502) construction
  line L400 (-10.3435, 11.1502) -> (-10.2123, 11.1327) construction
  line L401 (-10.2123, 11.1327) -> (-10.1491, 11.1113) construction
  line L402 (-10.1491, 11.1113) -> (-10.0277, 11.0415) construction
  line L403 (-10.0277, 11.0415) -> (-9.987, 10.9996) construction
  line L404 (-9.987, 10.9996) -> (-9.7959, 10.7903) construction
  line L405 (-9.7959, 10.7903) -> (-9.6645, 10.6176) construction
  line L406 (-9.6645, 10.6176) -> (-9.2615, 10.417) construction
  line L407 (-9.2615, 10.417) -> (-9.1006, 10.373) construction
  line L408 (-9.1006, 10.373) -> (-8.7708, 10.3489) construction
  line L409 (-8.7708, 10.3489) -> (-8.6052, 10.3692) construction
  line L410 (-8.6052, 10.3692) -> (-8.2593, 10.4826) construction
  line L411 (-8.2593, 10.4826) -> (-8.1332, 10.5728) construction
  line L412 (-8.1332, 10.5728) -> (-7.7864, 10.8269) construction
  line L413 (-7.7864, 10.8269) -> (-7.531, 10.9731) construction
  line L414 (-7.531, 10.9731) -> (-7.2442, 11.3181) construction
  line L415 (-7.2442, 11.3181) -> (-7.1645, 11.4638) construction
  line L416 (-7.1645, 11.4638) -> (-7.0649, 11.7786) construction
  line L417 (-7.0649, 11.7786) -> (-7.0464, 11.9445) construction
  line L418 (-7.0464, 11.9445) -> (-7.0704, 12.2323) construction
  line L419 (-7.0704, 12.2323) -> (-7.0969, 12.3919) construction
  line L420 (-7.0969, 12.3919) -> (-7.2878, 12.7615) construction
  line L421 (-7.2878, 12.7615) -> (-7.3995, 12.8796) construction
  line L422 (-7.3995, 12.8796) -> (-7.4328, 13.1225) construction
  line L423 (-7.4328, 13.1225) -> (-7.4289, 13.1891) construction
  line L424 (-7.4289, 13.1891) -> (-7.3972, 13.3113) construction
  line L425 (-7.3972, 13.3113) -> (-7.372, 13.3664) construction
  line L426 (-7.372, 13.3664) -> (-7.3034, 13.465) construction
  line L427 (-7.3034, 13.465) -> (-7.2607, 13.5079) construction
  line L428 (-7.2607, 13.5079) -> (-7.2114, 13.5423) construction
  arc A13 (-6.7172, 13.7941) -> (-7.2114, 13.5423) centre (0, 0) ccw
  spline S13 degree 3 poles (-6.7172, 13.7941) (-6.6546, 13.8158) (-6.5884, 13.8249) (-6.4563, 13.8174) (-6.3916, 13.8008) (-6.2723, 13.7436) (-6.2188, 13.7037) (-6.1249, 13.5999) (-6.0991, 13.5474) (-5.9821, 13.2893) (-5.9105, 13.0845) (-5.5892, 12.7691) (-5.4498, 12.6775) (-5.1435, 12.5527) (-4.9798, 12.5209) (-4.6158, 12.5218) (-4.468, 12.5686) (-4.0596, 12.7031) (-3.7715, 12.7632) (-3.3921, 13.0028) (-3.2713, 13.1166) (-3.0794, 13.3853) (-3.0104, 13.5374) (-2.9443, 13.8185) (-2.9203, 13.9785) (-2.9876, 14.3889) (-3.0573, 14.5358) (-3.0139, 14.7771) (-2.9896, 14.8393) (-2.9218, 14.9457) (-2.8807, 14.9902) (-2.7851, 15.0629) (-2.7312, 15.0904) (-2.6737, 15.108) knots 0 0 0 0 0.019863 0.019863 0.03972 0.03972 0.059573 0.059573 0.081705 0.081705 0.153115 0.153115 0.194508 0.194508 0.235922 0.235922 0.285548 0.285548 0.382717 0.382717 0.438735 0.438735 0.494976 0.494976 0.536961 0.536961 0.576712 0.576712 0.591396 0.591396 0.604738 0.604738 0.618079 0.618079 0.618079 0.618079
  line L429 (-6.7172, 13.7941) -> (-6.6546, 13.8158) construction
  line L430 (-6.6546, 13.8158) -> (-6.5884, 13.8249) construction
  line L431 (-6.5884, 13.8249) -> (-6.4563, 13.8174) construction
  line L432 (-6.4563, 13.8174) -> (-6.3916, 13.8008) construction
  line L433 (-6.3916, 13.8008) -> (-6.2723, 13.7436) construction
  line L434 (-6.2723, 13.7436) -> (-6.2188, 13.7037) construction
  line L435 (-6.2188, 13.7037) -> (-6.1249, 13.5999) construction
  line L436 (-6.1249, 13.5999) -> (-6.0991, 13.5474) construction
  line L437 (-6.0991, 13.5474) -> (-5.9821, 13.2893) construction
  line L438 (-5.9821, 13.2893) -> (-5.9105, 13.0845) construction
  line L439 (-5.9105, 13.0845) -> (-5.5892, 12.7691) construction
  line L440 (-5.5892, 12.7691) -> (-5.4498, 12.6775) construction
  line L441 (-5.4498, 12.6775) -> (-5.1435, 12.5527) construction
  line L442 (-5.1435, 12.5527) -> (-4.9798, 12.5209) construction
  line L443 (-4.9798, 12.5209) -> (-4.6158, 12.5218) construction
  line L444 (-4.6158, 12.5218) -> (-4.468, 12.5686) construction
  line L445 (-4.468, 12.5686) -> (-4.0596, 12.7031) construction
  line L446 (-4.0596, 12.7031) -> (-3.7715, 12.7632) construction
  line L447 (-3.7715, 12.7632) -> (-3.3921, 13.0028) construction
  line L448 (-3.3921, 13.0028) -> (-3.2713, 13.1166) construction
  line L449 (-3.2713, 13.1166) -> (-3.0794, 13.3853) construction
  line L450 (-3.0794, 13.3853) -> (-3.0104, 13.5374) construction
  line L451 (-3.0104, 13.5374) -> (-2.9443, 13.8185) construction
  line L452 (-2.9443, 13.8185) -> (-2.9203, 13.9785) construction
  line L453 (-2.9203, 13.9785) -> (-2.9876, 14.3889) construction
  line L454 (-2.9876, 14.3889) -> (-3.0573, 14.5358) construction
  line L455 (-3.0573, 14.5358) -> (-3.0139, 14.7771) construction
  line L456 (-3.0139, 14.7771) -> (-2.9896, 14.8393) construction
  line L457 (-2.9896, 14.8393) -> (-2.9218, 14.9457) construction
  line L458 (-2.9218, 14.9457) -> (-2.8807, 14.9902) construction
  line L459 (-2.8807, 14.9902) -> (-2.7851, 15.0629) construction
  line L460 (-2.7851, 15.0629) -> (-2.7312, 15.0904) construction
  line L461 (-2.7312, 15.0904) -> (-2.6737, 15.108) construction
  arc A14 (-2.1258, 15.1947) -> (-2.6737, 15.108) centre (0, 0) ccw
  spline S14 degree 3 poles (-2.1258, 15.1947) (-2.0596, 15.196) (-1.9938, 15.1842) (-1.8705, 15.1362) (-1.8141, 15.1004) (-1.7183, 15.0092) (-1.6797, 14.9547) (-1.6226, 14.827) (-1.6142, 14.7691) (-1.5827, 14.4874) (-1.5779, 14.2705) (-1.3697, 13.8713) (-1.2655, 13.7411) (-1.0128, 13.5278) (-0.8669, 13.4469) (-0.5204, 13.3353) (-0.3654, 13.3341) (0.0646, 13.3359) (0.3571, 13.304) (0.792, 13.4146) (0.942, 13.4856) (1.2076, 13.6817) (1.3202, 13.8051) (1.4699, 14.052) (1.5423, 14.1967) (1.605, 14.6079) (1.5841, 14.7691) (1.7, 14.9852) (1.7423, 15.0368) (1.8397, 15.1171) (1.8925, 15.1468) (2.0059, 15.1863) (2.0657, 15.1958) (2.1258, 15.1947) knots 0 0 0 0 0.019863 0.019863 0.03972 0.03972 0.059573 0.059573 0.081705 0.081705 0.153115 0.153115 0.194508 0.194508 0.235922 0.235922 0.285548 0.285548 0.382717 0.382717 0.438735 0.438735 0.494976 0.494976 0.536961 0.536961 0.576712 0.576712 0.591396 0.591396 0.604738 0.604738 0.618079 0.618079 0.618079 0.618079
  line L462 (-2.1258, 15.1947) -> (-2.0596, 15.196) construction
  line L463 (-2.0596, 15.196) -> (-1.9938, 15.1842) construction
  line L464 (-1.9938, 15.1842) -> (-1.8705, 15.1362) construction
  line L465 (-1.8705, 15.1362) -> (-1.8141, 15.1004) construction
  line L466 (-1.8141, 15.1004) -> (-1.7183, 15.0092) construction
  line L467 (-1.7183, 15.0092) -> (-1.6797, 14.9547) construction
  line L468 (-1.6797, 14.9547) -> (-1.6226, 14.827) construction
  line L469 (-1.6226, 14.827) -> (-1.6142, 14.7691) construction
  line L470 (-1.6142, 14.7691) -> (-1.5827, 14.4874) construction
  line L471 (-1.5827, 14.4874) -> (-1.5779, 14.2705) construction
  line L472 (-1.5779, 14.2705) -> (-1.3697, 13.8713) construction
  line L473 (-1.3697, 13.8713) -> (-1.2655, 13.7411) construction
  line L474 (-1.2655, 13.7411) -> (-1.0128, 13.5278) construction
  line L475 (-1.0128, 13.5278) -> (-0.8669, 13.4469) construction
  line L476 (-0.8669, 13.4469) -> (-0.5204, 13.3353) construction
  line L477 (-0.5204, 13.3353) -> (-0.3654, 13.3341) construction
  line L478 (-0.3654, 13.3341) -> (0.0646, 13.3359) construction
  line L479 (0.0646, 13.3359) -> (0.3571, 13.304) construction
  line L480 (0.3571, 13.304) -> (0.792, 13.4146) construction
  line L481 (0.792, 13.4146) -> (0.942, 13.4856) construction
  line L482 (0.942, 13.4856) -> (1.2076, 13.6817) construction
  line L483 (1.2076, 13.6817) -> (1.3202, 13.8051) construction
  line L484 (1.3202, 13.8051) -> (1.4699, 14.052) construction
  line L485 (1.4699, 14.052) -> (1.5423, 14.1967) construction
  line L486 (1.5423, 14.1967) -> (1.605, 14.6079) construction
  line L487 (1.605, 14.6079) -> (1.5841, 14.7691) construction
  line L488 (1.5841, 14.7691) -> (1.7, 14.9852) construction
  line L489 (1.7, 14.9852) -> (1.7423, 15.0368) construction
  line L490 (1.7423, 15.0368) -> (1.8397, 15.1171) construction
  line L491 (1.8397, 15.1171) -> (1.8925, 15.1468) construction
  line L492 (1.8925, 15.1468) -> (2.0059, 15.1863) construction
  line L493 (2.0059, 15.1863) -> (2.0657, 15.1958) construction
  line L494 (2.0657, 15.1958) -> (2.1258, 15.1947) construction
  arc A15 (2.6737, 15.108) -> (2.1258, 15.1947) centre (0, 0) ccw